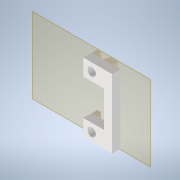
# Autodesk Inventor part: Voltera_Slide
Saved by Autodesk Inventor 2022 (Build 260153000, 153)
## iProperties
Created: 2022-08-22
Part Number: Voltera_Slide
Material: Generisch
Document SubType Name: Modeling
Designer: diederichbenedict
Density: 1 g/cm^3
Appearance: Vorgabe
Author: diederichbenedict
Autodesk Inventor part; units mm, degrees
ref_plane "YZ Plane" through (0, 0, 0) normal (1, 0, 0) x (0, 1, 0)
ref_plane "XZ Plane" through (0, 0, 0) normal (0, 1, 0) x (-1, 0, 0)
ref_plane "XY Plane" through (0, 0, 0) normal (0, 0, 1) x (1, 0, 0)
ref_plane "Arbeitsebene1" through (0, 0, 0) normal (0, 0, 1) x (1, 0, 0)
sketch "Skizze1" plane through (0, 0, 0) normal (0, 0, 1) x (1, 0, 0)
  line L0 (-4.8901, 59.5682) -> (-4.8901, -10.4318)
  line L1 (-22.7101, -0.4318) -> (-22.7101, 49.5682)
  line L2 (-16.7101, -0.4318) -> (-16.7101, 49.5682)
  circle A0 centre (-19.7101, 41.5682) radius 3 construction
  circle A1 centre (-19.7101, 3.6382) radius 3 construction
  line L3 (-25.7101, 47.5682) -> (-4.8901, 47.5682)
  line L4 (-4.8901, 47.5682) -> (-4.8901, 35.5682)
  line L5 (-4.8901, 35.5682) -> (-25.7101, 35.5682)
  line L6 (-25.7101, 35.5682) -> (-25.7101, 47.5682)
  line L7 (-4.8901, 9.6382) -> (-25.7101, 9.6382)
  line L8 (-25.7101, 9.6382) -> (-25.7101, -2.3618)
  line L9 (-25.7101, -2.3618) -> (-4.8901, -2.3618)
  line L10 (-4.8901, -2.3618) -> (-4.8901, 9.6382)
  circle A2 centre (-19.7101, 41.5682) radius 3.05
  circle A3 centre (-19.7101, 3.6382) radius 3.05
  line L11 (-4.8901, 35.5682) -> (-10.8901, 35.5682)
  line L12 (-10.8901, 35.5682) -> (-10.8901, 9.6382)
  line L13 (-10.8901, 9.6382) -> (-4.8901, 9.6382)
  line L14 (-4.8901, 9.6382) -> (-4.8901, 35.5682)
  point P0 (0, 0)
  point P1 (-4.8901, 47.5682)
  point P2 (-16.7101, 41.0182)
  point P3 (-22.7101, 41.0182)
  point P4 (-22.7101, 42.1182)
  point P5 (-16.7101, 42.1182)
  dimension "d0" = 6
  dimension "d1" = 3
  dimension "d2" = 6
  dimension "d3" = 37.93
  dimension "d4" = 8
  dimension "d5" = 6
  dimension "d6" = 6
  dimension "d7" = 6
  dimension "d8" = 6
  dimension "d9" = 6
  dimension "d10" = 6
  dimension "d11" = 6.1
  dimension "d12" = 6.1
  dimension "d13" = 6
  constraints: 30 end point, 6 parallel, 4 centre point, 3 horizontal, 3 perpendicular, 3 point on line, 3 vertical, 2 coincident, 6 other
  measures "d0" diameter of A0
  measures "d1" distance from line of A0.centre L2
  measures "d2" diameter of A1
  measures "d3" distance of A0.centre A1.centre
  measures "d4" vertical distance of L2.end A0.centre
  measures "d5" distance from line of A0.centre L3
  measures "d6" distance from line of L5 A0.centre
  measures "d7" distance from line of L6 A0.centre
  measures "d8" distance from line of A1.centre L7
  measures "d9" distance from line of L9 A1.centre
  measures "d10" distance from line of L8 A1.centre
  measures "d11" diameter of A2
  measures "d12" diameter of A3
  measures "d13" distance between parallel lines of L14 L12
extrude "Extrusion1" add sketch "Skizze1" along normal blind 6 contours L0 L5 L2 A2 L3 | L0 L7 L12 L5 | L2 A2 L1 L3 | L0 L9 L8 L7 L1 A3 L2 | A2 L2 | L1 A2 L5 L6 L3 | L5 L1 A2 L2 | L1 A2 | L2 A3 L1 L7
sketch "Skizze2" plane through (-25.7101, 47.5682, 0) normal (0, 1, 0) x (1, 0, 0)
  circle A0 centre (6, 3) radius 3 projected
  line L0 (0, 0) -> (0, 4)
  line L1 (0, 0) -> (4, 0) construction
  line L2 (0, 4) -> (2.6262, 4)
  line L3 (2.6262, 4) -> (3.698, 0)
  line L4 (0, 0) -> (14.82, 0) projected
  line L5 (9.3738, 4) -> (15.3738, 4)
  line L6 (15.3738, 4) -> (15.3738, 0)
  line L7 (15.3738, 0) -> (8.302, 0)
  line L8 (8.302, 0) -> (9.3738, 4)
  line L9 (30.8521, 0) -> (-5.142, 0) projected
  point P0 (25.7101, 0)
  point P1 (11.7707, 0)
  dimension "d16" = 4
  dimension "d17" = 90
  dimension "d18" = 15
  dimension "d19" = 15
  dimension "d22" = 6
  constraints: 16 end point, 4 perpendicular, 4 point on line, 2 tangent, 1 horizontal, 1 vertical
  measures "d16" distance of L0.start L0.end
  measures "d17" angle of L1 L0
  measures "d18" angle of L0 L3
  measures "d19" angle of L6 L8
  measures "d22" distance of L5.end L5.start
extrude "Extrusion2" add sketch "Skizze2" against normal up to surface (12 mm away) contours L3 L4 L0 L2 | L8 L5 L6 L7 L4
sketch "Skizze3" plane through (-25.7101, 9.6382, 0) normal (0, 1, 0) x (1, 0, 0)
  line L0 (20.82, 0) -> (15.3738, 0) projected
  line L1 (15.3738, 0) -> (15.3738, 4) projected
  line L2 (15.3738, 4) -> (9.3738, 4) projected
  line L3 (9.3738, 4) -> (8.302, 0) projected
  line L4 (8.302, 0) -> (3.698, 0) projected
  line L5 (3.698, 0) -> (2.6262, 4) projected
  line L6 (2.6262, 4) -> (0, 4) projected
  line L7 (0, 4) -> (0, -6) projected
  line L8 (20.82, -6) -> (0, -6) projected
  line L9 (20.82, 0) -> (20.82, -6) projected
  line L10 (0, 0) -> (0, -6) projected
  line L11 (0, 0) -> (3.698, 0)
  line L12 (8.302, 0) -> (15.3738, 0)
  point P0 (25.7101, 0)
  constraints: 4 end point, 1 collinear
extrude "Extrusion3" add sketch "Skizze3" against normal up to surface (12 mm away) contours L12 L3 L2 L1 | L11 L7 L6 L5
